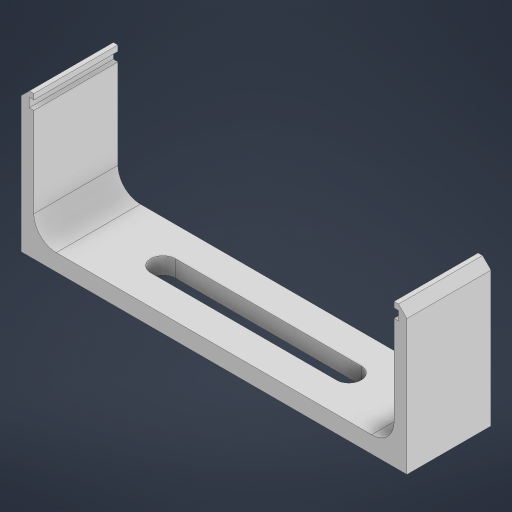
# Autodesk Inventor part: Discovery boar holder
Saved by Autodesk Inventor 2023 (Build 270158000, 158)
## iProperties
Created: 2024-01-04
Part Number: Discovery boar holder
Material: Generic
Document SubType Name: Modeling
Designer: nick_
Density: 1 g/cm^3
Appearance: Default
Author: nick_
Autodesk Inventor part; units mm, degrees
ref_plane "YZ Plane" through (0, 0, 0) normal (1, 0, 0) x (0, 1, 0)
ref_plane "XZ Plane" through (0, 0, 0) normal (0, 1, 0) x (-1, 0, 0)
ref_plane "XY Plane" through (0, 0, 0) normal (0, 0, 1) x (1, 0, 0)
sketch "Sketch1" plane through (0, 0, 0) normal (0, 0, 1) x (1, 0, 0)
  line L0 (0, 0) -> (-34.45, 0)
  line L1 (-34.45, 0) -> (-34.45, 25.6)
  line L2 (-34.45, 25.6) -> (-32.15, 25.6)
  line L3 (-32.15, 25.6) -> (-32.15, 24.6)
  line L4 (-32.15, 24.6) -> (-32.95, 24.6)
  line L5 (-32.95, 24.6) -> (-32.95, 23)
  line L6 (-32.95, 23) -> (-32.15, 23)
  line L7 (-32.15, 23) -> (-32.15, 3)
  line L8 (-32.15, 3) -> (0, 3)
  line L9 (0, 3) -> (0, 0)
  point P0 (-32.95, 23.8)
  point P1 (0, 1.5)
  dimension "d0" = 3
  dimension "d2" = 0.8
  dimension "d3" = 1
  dimension "d4" = 1.6
  dimension "d5" = 1.5
  dimension "d9" = 20
  dimension "d15" = 65.9
  constraints: 20 end point, 7 perpendicular, 2 midpoint, 1 horizontal, 1 parallel, 1 point on line, 1 vertical
  measures "d0" distance between parallel lines of L0 L8
  measures "d2" distance between parallel lines of L3 L5
  measures "d3" distance of L2.end L3.end
  measures "d4" distance of L4.end L5.end
  measures "d5" distance between parallel lines of L1 L5
  measures "d9" distance of L6.end L7.end
  measures "d15" diameter of L5 L9
extrude "Extrusion1" add sketch "Sketch1" along normal blind 15
mirror "Mirror1" about plane through (0, 0, 0) normal (1, 0, 0) of "Extrusion1"
sketch "Sketch2" plane through (-32.15, 3, 15) normal (0, 1, 0) x (1, 0, 0)
  line L0 (64.3, 15) -> (0, 15) construction
  line L1 (0, 15) -> (0, 0) construction
  line L2 (0, 0) -> (64.3, 0) construction
  line L3 (64.3, 15) -> (64.3, 0) construction
  line L4 (15.5721, 7.5) -> (48.7279, 7.5) construction
  line L5 (15.5721, 5.3) -> (48.7279, 5.3)
  line L6 (48.7279, 9.7) -> (15.5721, 9.7)
  arc A0 (15.5721, 9.7) -> (15.5721, 5.3) centre (15.5721, 7.5) ccw
  arc A1 (48.7279, 5.3) -> (48.7279, 9.7) centre (48.7279, 7.5) ccw
  line L7 (66.6, 15) -> (66.6, 0) projected
  point P0 (32.15, 15)
  point P1 (32.15, 7.5)
  point P2 (32.15, 15)
  point P3 (66.6, 7.5)
  dimension "d12" = 2.2
  constraints: 8 end point, 4 point on circle, 4 tangent, 3 midpoint, 2 centre point, 2 parallel, 1 horizontal alignment, 1 vertical alignment
  measures "d12" radius of A0
extrude "Extrusion2" cut sketch "Sketch2" against normal through all
chamfer "Chamfer1" distance 1.5 angle 45 2 edges at (-34.45, 25.6, 7.5) (34.45, 25.6, 7.5)
fillet "Fillet1" radius 4 2 edges at (32.15, 3, 7.5) (-32.15, 3, 7.5)
body "Solid1"
